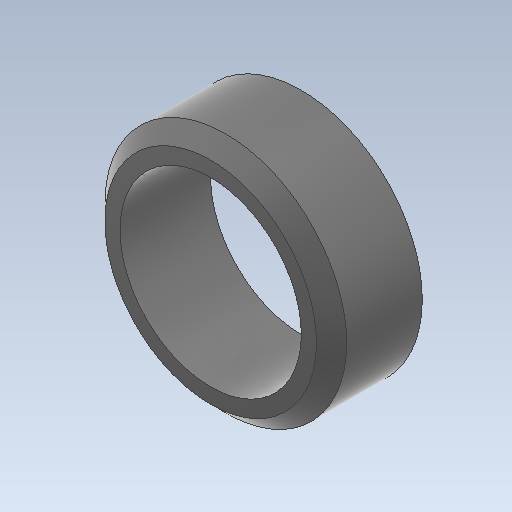
# Autodesk Inventor part: オイレス6-10
Saved by Autodesk Inventor 2020.4 (Build 244396000, 396)
## iProperties
Created: 2020-02-11
Part Number: オイレス6-10
Material: アセタール樹脂、黒
Document SubType Name: Modeling
Designer: happy
Density: 1.425 g/cm^3
Appearance: 滑らか - 黒
Mass: 0.0897219 g
Surface Area: 1.68243 cm^2
Volume: 0.0629628 cm^3
Author: happy
Autodesk Inventor part; units mm, degrees
ref_plane "YZ Plane" through (0, 0, 0) normal (1, 0, 0) x (0, 1, 0)
ref_plane "XZ Plane" through (0, 0, 0) normal (0, 1, 0) x (-1, 0, 0)
sketch "スケッチ1" plane through (0, 0, 0) normal (0, 0, 1) x (1, 0, 0)
  circle A0 centre (0, 0) radius 5.5
  circle A1 centre (0, 0) radius 3
  dimension "d0" = 11
  dimension "d1" = 6
  constraints: 2 centre point, 2 coincident
  measures "d0" diameter of A0
  measures "d1" diameter of A1
ref_plane "作業平面1" through (0, 0, 1) normal (0, 0, 1) x (1, 0, 0)
sketch "スケッチ2" plane through (0, 0, 1) normal (0, 0, 1) x (1, 0, 0)
  circle A0 centre (0, 0) radius 4
  circle A1 centre (0, 0) radius 3
  dimension "d4" = 8
  constraints: 2 centre point, 1 coincident, 2 other
  measures "d4" diameter of A0
extrude "押し出し2" add sketch "スケッチ2" along normal blind 3
chamfer "面取り2" distance 0.5 angle 45 1 edges at (-4, 0, 4)
